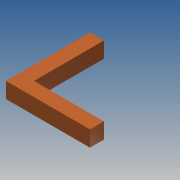
# Autodesk Inventor part: bench
Saved by Autodesk Inventor 2013 (Build 170138000, 138)
## iProperties
Created: 2014-01-02
Part Number: bench
Material: Wood (Cherry)
Document SubType Name: Modeling
Designer: ddeboer
Mass: 646044 g
Surface Area: 105703 cm^2
Volume: 1.29209e+06 cm^3
Density: 0.5 g/cm^3
Author: ddeboer
Autodesk Inventor part; units mm, degrees
ref_plane "YZ Plane" through (0, 0, 0) normal (1, 0, 0) x (0, 1, 0)
ref_plane "XZ Plane" through (0, 0, 0) normal (0, 1, 0) x (-1, 0, 0)
ref_plane "XY Plane" through (0, 0, 0) normal (0, 0, 1) x (1, 0, 0)
sketch "Sketch1" plane through (0, 0, 0) normal (0, 1, 0) x (-1, 0, 0)
  line L0 (0, 0) -> (-2438.4, 0)
  line L1 (0, 0) -> (0, -2438.4)
  line L2 (-2438.4, -406.4) -> (-406.4, -406.4)
  line L3 (-406.4, -406.4) -> (-406.4, -2438.4)
  line L4 (-2438.4, -406.4) -> (-2438.4, 0)
  line L5 (-406.4, -2438.4) -> (0, -2438.4)
  dimension "d0" = 2438.4
  dimension "d2" = 2438.4
  dimension "d3" = 406.4
  constraints: 12 end point, 3 perpendicular, 1 horizontal, 1 parallel, 1 other
  measures "d0" distance of L0.start L0.end
  measures "d2" distance of L0.start L1.end
  measures "d3" distance between parallel lines of L2 L0
extrude "Extrusion1" add sketch "Sketch1" along normal blind 457.2
body "Solid1"
